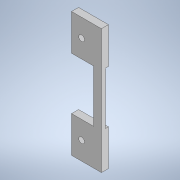
# Autodesk Inventor part: imu_cable_holder
Saved by Autodesk Inventor 2021 (Build 250183000, 183)
## iProperties
Created: 2021-01-13
Part Number: imu_cable_holder
Material: Generic
Document SubType Name: Modeling
Designer: Mateusz
Density: 1 g/cm^3
Appearance: Default
Author: Mateusz
Autodesk Inventor part; units mm, degrees
ref_plane "YZ Plane" through (0, 0, 0) normal (1, 0, 0) x (0, 1, 0)
ref_plane "XZ Plane" through (0, 0, 0) normal (0, 1, 0) x (-1, 0, 0)
ref_plane "XY Plane" through (0, 0, 0) normal (0, 0, 1) x (1, 0, 0)
sketch "Sketch1" plane through (0, 0, 0) normal (0, 0, 1) x (1, 0, 0)
  circle A0 centre (14.9935, -706.254) radius 1.4499
  circle A1 centre (14.9932, -750.254) radius 1.4502
  line L0 (24.8521, -741.254) -> (24.8525, -697.2541) projected
  line L1 (24.8519, -759.254) -> (24.8521, -741.254) projected
  line L2 (20.3016, -715.254) -> (14.3016, -715.254) projected
  line L3 (9.9969, -697.2539) -> (24.8525, -697.2541)
  line L4 (24.8525, -697.2541) -> (24.8527, -715.2539)
  line L5 (24.8527, -715.2539) -> (24.8527, -715.2539)
  line L6 (24.8521, -741.254) -> (9.9968, -741.2539)
  line L7 (9.9968, -741.2539) -> (9.9968, -759.2539)
  line L8 (9.9968, -759.2539) -> (24.8519, -759.254)
  line L9 (24.8519, -759.254) -> (24.8521, -741.254)
  line L10 (24.8527, -715.2539) -> (9.9968, -715.2538)
  line L11 (9.9969, -697.2539) -> (9.9968, -715.2538)
  line L12 (24.8527, -715.2539) -> (24.8521, -741.254)
  line L13 (24.8521, -741.254) -> (20.8521, -741.254)
  line L14 (20.8521, -741.254) -> (20.8522, -715.2538)
  point P0 (0, 0)
  point P1 (24.8523, -715.2539)
  constraints: 24 end point, 2 centre point, 2 perpendicular, 2 point on line, 1 collinear
extrude "Extrusion1" add sketch "Sketch1" along normal blind 2
sketch "Sketch3" plane through (0, 0, 2) normal (0, 0, 1) x (1, 0, 0)
  line L0 (9.9968, -715.2538) -> (20.8522, -715.2538) projected
  line L1 (20.8522, -715.2538) -> (20.8521, -741.254) projected
  line L2 (20.8521, -741.254) -> (9.9968, -741.2539) projected
  line L3 (9.9968, -741.2539) -> (9.9968, -759.2539) projected
  line L4 (9.9968, -759.2539) -> (24.8519, -759.254) projected
  line L5 (24.8519, -759.254) -> (24.8525, -697.2541) projected
  line L6 (24.8525, -697.2541) -> (9.9969, -697.2539) projected
  line L7 (9.9969, -697.2539) -> (9.9968, -715.2538) projected
  circle A0 centre (14.9935, -706.254) radius 1.4499 projected
  circle A1 centre (14.9932, -750.254) radius 1.4502 projected
  line L8 (9.9968, -715.2538) -> (20.8522, -715.2538) projected
  line L9 (20.8522, -715.2538) -> (24.8523, -715.2538)
  line L10 (24.8519, -759.254) -> (24.8525, -697.2541) projected
  line L11 (20.8522, -715.2538) -> (20.8521, -741.254) projected
  line L12 (20.8521, -741.254) -> (24.8521, -741.254)
  point P0 (0, 0)
  constraints: 4 end point, 2 point on line, 1 horizontal, 1 parallel
extrude "Extrusion3" add sketch "Sketch3" along normal blind 1.5 contours L7 L6 L5 L9 L0 | L12 L5 L4 L3 L2
body "Solid1"
